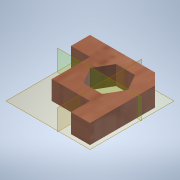
# Autodesk Inventor part: bevestiging deksel
Saved by Autodesk Inventor 2021 (Build 250183000, 183)
## iProperties
Manager: Pierloot J.
Company: Emmaüs Bovenbouw Aalter
Created: 2021-01-26
Part Number: bevestiging deksel
Material: S235
Catalog Web Link: http://emmausbovenbouw.op-weg.be/
Vendor: Emmaüsinstituut Bovenbouw Aalter
Document SubType Name: Modeling
Designer: iskhak.tchuytiyev
Engineer: Pierloot J.
Manufacturer: Standard
Standards Organization: Custom
Density: 7.86 g/cm^3
Appearance: White Oak - Natural Medium Gloss
Title: Algemene titel
Subject: Specifieke titel
Author: iskhak.tchuytiyev
Keywords: Ruwe Ø xxxxx
Comments: Opmerking
Autodesk Inventor part; units mm, degrees
sketch "Sketch1" plane through (0, 0, 0) normal (0, 0, 1) x (1, 0, 0)
  line L0 (0, 2.8582) -> (0, -2.8582) construction
  line L1 (-5.7775, 0) -> (5.7775, 0) construction
  point P0 (0, 0)
  point P1 (0, 0)
  constraints: 4 end point, 2 midpoint, 1 coincident, 1 horizontal, 1 vertical
sketch "Sketch2" plane through (0, 0, 0) normal (0, 0, 1) x (1, 0, 0)
  line L0 (2.4826, 4.3) -> (4.9652, 0)
  line L1 (4.9652, 0) -> (2.4826, -4.3)
  line L2 (2.4826, -4.3) -> (-2.4826, -4.3)
  line L3 (-2.4826, -4.3) -> (-4.9652, 0)
  line L4 (-4.9652, 0) -> (-2.4826, 4.3)
  line L5 (-2.4826, 4.3) -> (2.4826, 4.3)
  line L6 (-7.5, 7.5) -> (7.5, 7.5)
  line L7 (7.5, 7.5) -> (7.5, -7.5)
  line L8 (7.5, -7.5) -> (-7.5, -7.5)
  line L9 (-7.5, -7.5) -> (-7.5, 7.5)
  line L10 (-7.5, 7.5) -> (7.5, -7.5) construction
  line L11 (7.5, 7.5) -> (-7.5, -7.5) construction
  point P0 (0, 0)
  point P1 (0, 0)
  dimension "d0" = 8.6
  dimension "d1" = 15
  dimension "d2" = 15
  constraints: 24 end point, 2 midpoint, 2 parallel, 1 coincident, 1 horizontal, 1 perpendicular, 13 other
  measures "d0" distance between parallel lines of L5 L2
  measures "d1" distance of L7.end L8.end
  measures "d2" distance of L6.end L7.end
extrude "Extrusion1" add sketch "Sketch2" along normal blind 5
chamfer "Chamfer1" distance 3 angle 45 1 edges at (7.5, 7.5, 2.5)
sketch "Sketch3" plane through (-7.5, -7.5, 0) normal (-1, 0, 0) x (0, 0, 1)
  line L0 (0, 15) -> (5, 15)
  line L1 (5, 15) -> (5, 10)
  line L2 (5, 10) -> (0, 10)
  line L3 (0, 10) -> (0, 15)
  point P0 (0, 7.5)
  dimension "d8" = 5
  dimension "d9" = 5
  constraints: 8 end point, 2 parallel, 1 horizontal, 1 perpendicular
  measures "d8" distance of L1.end L2.end
  measures "d9" distance of L0.end L1.end
extrude "Extrusion2" add sketch "Sketch3" along normal blind 5
sketch "Sketch4" plane through (-7.5, -7.5, 0) normal (0, -1, 0) x (1, 0, 0)
  line L0 (15, 0) -> (15, 5) projected
  line L1 (15, 5) -> (10, 5)
  line L2 (10, 5) -> (10, 0)
  line L3 (10, 0) -> (15, 0)
  line L4 (15, 0) -> (15, 5)
  point P0 (7.5, 0)
  dimension "d12" = 5
  dimension "d13" = 5
  constraints: 8 end point, 2 parallel, 1 horizontal, 1 perpendicular
  measures "d12" distance of L3.end L2.end
  measures "d13" distance of L2.end L1.end
extrude "Extrusion3" add sketch "Sketch4" along normal blind 5
body "Solid1"
